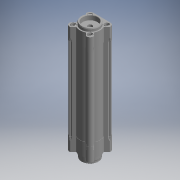
# Autodesk Inventor part: ESBF-BS-40-100---(ZR_-_-)
Saved by Autodesk Inventor 2017.3 (Build 213256000, 256)
## iProperties
Part Number: ESBF-BS-40-100---(ZR_-_-)
Material: Generic
Catalog Web Link: www.cadenas.de
Description: ESBF-(ZR)-Electro-cylinder
Vendor: FESTO
Document SubType Name: Modeling
Designer: partserver
Manufacturer: FESTO
Mass: 374.092 g
Surface Area: 1016.03 cm^2
Volume: 374.092 cm^3
Density: 1 g/cm^3
Appearance: PSOLRGB-192-192-192
Category: PARTsolutions
Company: FESTO
Title: ESBF-BS-40-100---(ZR_-_-)
Author: Cadenas PARTsolutions
Comments: Electro-cylinder
PSOL_IDENT_0: {$CADENAS_DATA\23d-libs\festo\parts\e\esbf\parts\esbf_zr.prj},208 {VTYP=3D},{NB=ESBF-BS-40-100---(ZR
PSOL_IDENT_1: _-_-)},{LINA=ESBF-BS-40-100---(ZR_-_-)},{NN=ESBF-(ZR)},{DATE=27.05.2021 13:20:18},{GEOMDATE=27.05.20
PSOL_IDENT_2: 21 13:19:59},{VERSION=},{LINEID=50},{WBVAR=HUB,SCEL,BWE},{WBNUMERIC=HUB}  {NB=ESBF-BS-40-100---(ZR_-
PSOL_IDENT_3: _-)},{LINA=ESBF-BS-40-100---(ZR_-_-)},{KT=DUMMY},{TNR=8022585},{TYP=ESBF-BS-40},{KDM=40},{HUB=100},{
PSOL_IDENT_4: SCEL=-},{BWE=-},{A=-6.000},{ANG=40.000},{B=39.000},{B1=38.000},{BE1=10.000},{BG=16.000},{D1=24.000},
PSOL_IDENT_5: {D2=8.000},{D2R=9.000},{D3=40.000},{D3R=10.500},{D5=33.000},{E=54.000},{E1=0.000},{EG=11.500},{G=30.
PSOL_IDENT_6: 000},{G1=30.000},{HE=2.100},{R1=8.000},{R1I=7.500},{R2=45.300},{TG=38.000},{RI=22.250},{RK=1.800},{T
PSOL_IDENT_7: 5=10.200},{J2=0.000},{L10=13.000},{L14=21.100},{L16=18.700},{L18=5.500},{L1=14.000},{L2=144.000},{L3=
PSOL_IDENT_8: 18.400},{L7=24.000},{M1=6.000},{PL=0.000},{SW3=6.000},{SWT=4.000},{VA=7.000},{VD=9.000},{D100=7.000}
PSOL_IDENT_9: ,{GUA=10.000},{B2=4.000},{D6=25.500},{D7=35.200},{BWE1='-','F1A'}
NB: ESBF-BS-40-100---(ZR_-_-)
NN: ESBF-(ZR)
NT: Electro-cylinder
NBSYN: $TYP.-$HUB.---(ZR_$SCEL._$BWE.)
LINA: ESBF-BS-40-100---(ZR_-_-)
CATALOG: Festo
TNR: 8022585
TYP: ESBF-BS-40
KDM: 40
HUB: 100
SCEL: -
BWE: -
A: -6
ANG: 40
B: 39
B1: 38
BE1: 10
BG: 16
D1: 24
D2: 8
D2R: 9
D3: 40
D3R: 10.5
D5: 33
E: 54
E1: 0
EG: 11.5
G: 30
G1: 30
HE: 2.1
R1: 8
R1I: 7.5
R2: 45.3
TG: 38
RI: 22.25
RK: 1.8
T5: 10.2
J2: 0
L10: 13
L14: 21.1
L16: 18.7
L18: 5.5
L1: 14
L2: 144
L3: 18.4
L7: 24
M1: 6
PL: 0
SW3: 6
SWT: 4
VA: 7
VD: 9
D100: 7
GUA: 10
B2: 4
D6: 25.5
D7: 35.2
SUPPLIER: FESTO
ARTICLENO: ESBF-BS-40-100---(ZR_-_-)
BOMINFO: ESBF-BS-40-100---(ZR_-_-)
CREATOR: CADENAS GmbH
Autodesk Inventor part; units mm, degrees
sketch "Sketch_1" plane through (0, 0, -30) normal (0, 0, 1) x (1, 0, 0)
  arc A0 (-27, 18.2218) -> (-26.7071, 17.5147) centre (-26, 18.2218) ccw
  line L0 (-26.7071, 17.5147) -> (-20.4561, 11.2637)
  arc A1 (-20.2683, 10.1102) -> (-20.4561, 11.2637) centre (-21.1632, 10.5566) ccw
  arc A2 (-20.2683, 10.1102) -> (-20.2683, -10.1102) centre (0, 0) ccw
  arc A3 (-20.4561, -11.2637) -> (-20.2683, -10.1102) centre (-21.1632, -10.5566) ccw
  line L1 (-20.4561, -11.2637) -> (-26.7071, -17.5147)
  arc A4 (-26.7071, -17.5147) -> (-27, -18.2218) centre (-26, -18.2218) ccw
  line L2 (-27, -18.2218) -> (-27, -19)
  arc A5 (-27, -19) -> (-19, -27) centre (-19, -19) ccw
  line L3 (-19, -27) -> (-18.2218, -27)
  arc A6 (-18.2218, -27) -> (-17.5147, -26.7071) centre (-18.2218, -26) ccw
  line L4 (-17.5147, -26.7071) -> (-11.2637, -20.4561)
  arc A7 (-10.1102, -20.2683) -> (-11.2637, -20.4561) centre (-10.5566, -21.1632) ccw
  arc A8 (-10.1102, -20.2683) -> (10.1102, -20.2683) centre (0, 0) ccw
  arc A9 (11.2637, -20.4561) -> (10.1102, -20.2683) centre (10.5566, -21.1632) ccw
  line L5 (11.2637, -20.4561) -> (17.5147, -26.7071)
  arc A10 (17.5147, -26.7071) -> (18.2218, -27) centre (18.2218, -26) ccw
  line L6 (18.2218, -27) -> (19, -27)
  arc A11 (19, -27) -> (27, -19) centre (19, -19) ccw
  line L7 (27, -19) -> (27, -18.2218)
  arc A12 (27, -18.2218) -> (26.7071, -17.5147) centre (26, -18.2218) ccw
  line L8 (26.7071, -17.5147) -> (20.4561, -11.2637)
  arc A13 (20.2683, -10.1102) -> (20.4561, -11.2637) centre (21.1632, -10.5566) ccw
  arc A14 (20.2683, -10.1102) -> (20.2683, 10.1102) centre (0, 0) ccw
  arc A15 (20.4561, 11.2637) -> (20.2683, 10.1102) centre (21.1632, 10.5566) ccw
  line L9 (20.4561, 11.2637) -> (26.7071, 17.5147)
  arc A16 (26.7071, 17.5147) -> (27, 18.2218) centre (26, 18.2218) ccw
  line L10 (27, 18.2218) -> (27, 19)
  arc A17 (27, 19) -> (19, 27) centre (19, 19) ccw
  line L11 (19, 27) -> (-19, 27)
  arc A18 (-19, 27) -> (-27, 19) centre (-19, 19) ccw
  line L12 (-27, 19) -> (-27, 18.2218)
  constraints: 38 point on circle, 26 end point, 19 centre point
extrude "Extrusion1" add sketch "Sketch_1" along normal blind 30
sketch "Sketch_8" plane through (0, 0, -30) normal (0, 0, 1) x (1, 0, 0)
  line L0 (-50, 45) -> (50, 45)
  line L1 (-19.3, 33.75) -> (-19.3, 27)
  line L2 (-19.3, 27) -> (-18.203, 25.1)
  arc A0 (-18.203, 25.1) -> (-18.0298, 25) centre (-18.0298, 25.2) ccw
  line L3 (-18.0298, 25) -> (-17.3281, 25)
  arc A1 (-17.3281, 25) -> (-17.1867, 25.0586) centre (-17.3281, 25.2) ccw
  line L4 (-17.1867, 25.0586) -> (-15.2453, 27)
  line L5 (-15.2453, 27) -> (15.2453, 27)
  line L6 (15.2453, 27) -> (17.1867, 25.0586)
  arc A2 (17.1867, 25.0586) -> (17.3281, 25) centre (17.3281, 25.2) ccw
  line L7 (17.3281, 25) -> (18.0298, 25)
  arc A3 (18.0298, 25) -> (18.203, 25.1) centre (18.0298, 25.2) ccw
  line L8 (18.203, 25.1) -> (19.3, 27)
  line L9 (19.3, 27) -> (19.3, 33.75)
  line L10 (19.3, 33.75) -> (-19.3, 33.75)
  constraints: 22 end point, 8 point on circle, 4 centre point
revolve "Revolution1" cut sketch "Sketch_8" angle 360 about axis through (-50, 45, -30) along (-1, 0, 0)
sketch "Sketch_21" plane through (0, 0, -30) normal (0, 0, 1) x (1, 0, 0)
  line L0 (50, -45) -> (-50, -45)
  line L1 (-19.3, -33.75) -> (19.3, -33.75)
  line L2 (19.3, -33.75) -> (19.3, -27)
  line L3 (19.3, -27) -> (18.203, -25.1)
  arc A0 (18.203, -25.1) -> (18.0298, -25) centre (18.0298, -25.2) ccw
  line L4 (18.0298, -25) -> (5.7378, -25)
  arc A1 (-5.7378, -25) -> (5.7378, -25) centre (0, 0) ccw
  line L5 (-5.7378, -25) -> (-18.0298, -25)
  arc A2 (-18.0298, -25) -> (-18.203, -25.1) centre (-18.0298, -25.2) ccw
  line L6 (-18.203, -25.1) -> (-19.3, -27)
  line L7 (-19.3, -27) -> (-19.3, -33.75)
  constraints: 16 end point, 6 point on circle, 3 centre point
revolve "Revolution2" cut sketch "Sketch_21" angle 360 about axis through (50, -45, -30) along (1, 0, 0)
sketch "Sketch_23" plane through (0, 0, -30) normal (0, 0, 1) x (1, 0, 0)
  line L0 (45, 50) -> (45, -50)
  line L1 (25, -5.7378) -> (25, -18.0298)
  arc A0 (25, -18.0298) -> (25.1, -18.203) centre (25.2, -18.0298) ccw
  line L2 (25.1, -18.203) -> (27, -19.3)
  line L3 (27, -19.3) -> (33.75, -19.3)
  line L4 (33.75, -19.3) -> (33.75, 19.3)
  line L5 (33.75, 19.3) -> (27, 19.3)
  line L6 (27, 19.3) -> (25.1, 18.203)
  arc A1 (25.1, 18.203) -> (25, 18.0298) centre (25.2, 18.0298) ccw
  line L7 (25, 18.0298) -> (25, 5.7378)
  arc A2 (25, -5.7378) -> (25, 5.7378) centre (0, 0) ccw
  constraints: 16 end point, 6 point on circle, 3 centre point
revolve "Revolution3" cut sketch "Sketch_23" angle 360 about axis through (45, 50, -30) along (0, 1, 0)
sketch "Sketch_24" plane through (0, 0, -30) normal (0, 0, 1) x (1, 0, 0)
  line L0 (-45, -50) -> (-45, 50)
  line L1 (-33.75, -19.3) -> (-27, -19.3)
  line L2 (-27, -19.3) -> (-25.1, -18.203)
  arc A0 (-25.1, -18.203) -> (-25, -18.0298) centre (-25.2, -18.0298) ccw
  line L3 (-25, -18.0298) -> (-25, -5.7378)
  arc A1 (-25, 5.7378) -> (-25, -5.7378) centre (0, 0) ccw
  line L4 (-25, 5.7378) -> (-25, 18.0298)
  arc A2 (-25, 18.0298) -> (-25.1, 18.203) centre (-25.2, 18.0298) ccw
  line L5 (-25.1, 18.203) -> (-27, 19.3)
  line L6 (-27, 19.3) -> (-33.75, 19.3)
  line L7 (-33.75, 19.3) -> (-33.75, -19.3)
  constraints: 16 end point, 6 point on circle, 3 centre point
revolve "Revolution4" cut sketch "Sketch_24" angle 360 about axis through (-45, -50, -30) along (0, -1, 0)
sketch "Sketch_41" plane through (0, 0, 0) normal (1, 0, 0) x (0, 1, 0)
  line L0 (0, -214) -> (0, -30)
  line L1 (0, -30) -> (5, -30)
  line L2 (5, -30) -> (5, -214)
  line L3 (5, -214) -> (0, -214)
  line L4 (0, -214) -> (0, -30)
  constraints: 10 end point
revolve "Revolution5" add sketch "Sketch_41" angle 360 about axis through (0, 0, -214) along (0, 0, -1)
sketch "Sketch_5" plane through (0, 0, -214) normal (0, 0, 1) x (1, 0, 0)
  arc A0 (-27, 18.2218) -> (-26.7071, 17.5147) centre (-26, 18.2218) ccw
  line L0 (-26.7071, 17.5147) -> (-20.4561, 11.2637)
  arc A1 (-20.2683, 10.1102) -> (-20.4561, 11.2637) centre (-21.1632, 10.5566) ccw
  arc A2 (-20.2683, 10.1102) -> (-20.2683, -10.1102) centre (0, 0) ccw
  arc A3 (-20.4561, -11.2637) -> (-20.2683, -10.1102) centre (-21.1632, -10.5566) ccw
  line L1 (-20.4561, -11.2637) -> (-26.7071, -17.5147)
  arc A4 (-26.7071, -17.5147) -> (-27, -18.2218) centre (-26, -18.2218) ccw
  line L2 (-27, -18.2218) -> (-27, -19)
  arc A5 (-27, -19) -> (-19, -27) centre (-19, -19) ccw
  line L3 (-19, -27) -> (-18.2218, -27)
  arc A6 (-18.2218, -27) -> (-17.5147, -26.7071) centre (-18.2218, -26) ccw
  line L4 (-17.5147, -26.7071) -> (-11.2637, -20.4561)
  arc A7 (-10.1102, -20.2683) -> (-11.2637, -20.4561) centre (-10.5566, -21.1632) ccw
  arc A8 (-10.1102, -20.2683) -> (10.1102, -20.2683) centre (0, 0) ccw
  arc A9 (11.2637, -20.4561) -> (10.1102, -20.2683) centre (10.5566, -21.1632) ccw
  line L5 (11.2637, -20.4561) -> (17.5147, -26.7071)
  arc A10 (17.5147, -26.7071) -> (18.2218, -27) centre (18.2218, -26) ccw
  line L6 (18.2218, -27) -> (19, -27)
  arc A11 (19, -27) -> (27, -19) centre (19, -19) ccw
  line L7 (27, -19) -> (27, -18.2218)
  arc A12 (27, -18.2218) -> (26.7071, -17.5147) centre (26, -18.2218) ccw
  line L8 (26.7071, -17.5147) -> (20.4561, -11.2637)
  arc A13 (20.2683, -10.1102) -> (20.4561, -11.2637) centre (21.1632, -10.5566) ccw
  arc A14 (20.2683, -10.1102) -> (20.2683, 10.1102) centre (0, 0) ccw
  arc A15 (20.4561, 11.2637) -> (20.2683, 10.1102) centre (21.1632, 10.5566) ccw
  line L9 (20.4561, 11.2637) -> (26.7071, 17.5147)
  arc A16 (26.7071, 17.5147) -> (27, 18.2218) centre (26, 18.2218) ccw
  line L10 (27, 18.2218) -> (27, 19)
  arc A17 (27, 19) -> (19, 27) centre (19, 19) ccw
  line L11 (19, 27) -> (-19, 27)
  arc A18 (-19, 27) -> (-27, 19) centre (-19, 19) ccw
  line L12 (-27, 19) -> (-27, 18.2218)
  constraints: 38 point on circle, 26 end point, 19 centre point
extrude "Extrusion2" add sketch "Sketch_5" against normal blind 30
sketch "Sketch_4" plane through (0, 0, -214) normal (0, 0, 1) x (1, 0, 0)
  line L0 (-50, 45) -> (50, 45)
  line L1 (-19.3, 33.75) -> (-19.3, 27)
  line L2 (-19.3, 27) -> (-18.203, 25.1)
  arc A0 (-18.203, 25.1) -> (-18.0298, 25) centre (-18.0298, 25.2) ccw
  line L3 (-18.0298, 25) -> (-17.3281, 25)
  arc A1 (-17.3281, 25) -> (-17.1867, 25.0586) centre (-17.3281, 25.2) ccw
  line L4 (-17.1867, 25.0586) -> (-15.2453, 27)
  line L5 (-15.2453, 27) -> (15.2453, 27)
  line L6 (15.2453, 27) -> (17.1867, 25.0586)
  arc A2 (17.1867, 25.0586) -> (17.3281, 25) centre (17.3281, 25.2) ccw
  line L7 (17.3281, 25) -> (18.0298, 25)
  arc A3 (18.0298, 25) -> (18.203, 25.1) centre (18.0298, 25.2) ccw
  line L8 (18.203, 25.1) -> (19.3, 27)
  line L9 (19.3, 27) -> (19.3, 33.75)
  line L10 (19.3, 33.75) -> (-19.3, 33.75)
  constraints: 22 end point, 8 point on circle, 4 centre point
revolve "Revolution6" cut sketch "Sketch_4" angle 360 about axis through (-50, 45, -214) along (-1, 0, 0)
sketch "Sketch_25" plane through (0, 0, -214) normal (0, 0, 1) x (1, 0, 0)
  line L0 (50, -45) -> (-50, -45)
  line L1 (-19.3, -27) -> (-19.3, -36)
  line L2 (-19.3, -36) -> (19.3, -36)
  line L3 (19.3, -36) -> (19.3, -27)
  line L4 (19.3, -27) -> (18.203, -25.1)
  arc A0 (18.203, -25.1) -> (18.0298, -25) centre (18.0298, -25.2) ccw
  line L5 (18.0298, -25) -> (5.7378, -25)
  arc A1 (-5.7378, -25) -> (5.7378, -25) centre (0, 0) ccw
  line L6 (-5.7378, -25) -> (-18.0298, -25)
  arc A2 (-18.0298, -25) -> (-18.203, -25.1) centre (-18.0298, -25.2) ccw
  line L7 (-18.203, -25.1) -> (-19.3, -27)
  constraints: 16 end point, 6 point on circle, 3 centre point
revolve "Revolution7" cut sketch "Sketch_25" angle 360 about axis through (50, -45, -214) along (1, 0, 0)
sketch "Sketch_26" plane through (0, 0, -214) normal (0, 0, 1) x (1, 0, 0)
  line L0 (45, 50) -> (45, -50)
  line L1 (25, -5.7378) -> (25, -18.0298)
  arc A0 (25, -18.0298) -> (25.1, -18.203) centre (25.2, -18.0298) ccw
  line L2 (25.1, -18.203) -> (27, -19.3)
  line L3 (27, -19.3) -> (33.75, -19.3)
  line L4 (33.75, -19.3) -> (33.75, 19.3)
  line L5 (33.75, 19.3) -> (27, 19.3)
  line L6 (27, 19.3) -> (25.1, 18.203)
  arc A1 (25.1, 18.203) -> (25, 18.0298) centre (25.2, 18.0298) ccw
  line L7 (25, 18.0298) -> (25, 5.7378)
  arc A2 (25, -5.7378) -> (25, 5.7378) centre (0, 0) ccw
  constraints: 16 end point, 6 point on circle, 3 centre point
revolve "Revolution8" cut sketch "Sketch_26" angle 360 about axis through (45, 50, -214) along (0, 1, 0)
sketch "Sketch_27" plane through (0, 0, -214) normal (0, 0, 1) x (1, 0, 0)
  line L0 (-45, -50) -> (-45, 50)
  line L1 (-33.75, -19.3) -> (-27, -19.3)
  line L2 (-27, -19.3) -> (-25.1, -18.203)
  arc A0 (-25.1, -18.203) -> (-25, -18.0298) centre (-25.2, -18.0298) ccw
  line L3 (-25, -18.0298) -> (-25, -5.7378)
  arc A1 (-25, 5.7378) -> (-25, -5.7378) centre (0, 0) ccw
  line L4 (-25, 5.7378) -> (-25, 18.0298)
  arc A2 (-25, 18.0298) -> (-25.1, 18.203) centre (-25.2, 18.0298) ccw
  line L5 (-25.1, 18.203) -> (-27, 19.3)
  line L6 (-27, 19.3) -> (-33.75, 19.3)
  line L7 (-33.75, 19.3) -> (-33.75, -19.3)
  constraints: 16 end point, 6 point on circle, 3 centre point
revolve "Revolution9" cut sketch "Sketch_27" angle 360 about axis through (-45, -50, -214) along (0, -1, 0)
sketch "Sketch_43" plane through (0, 0, -30) normal (0, 0, 1) x (1, 0, 0)
  arc A0 (-26.5208, -19.5466) -> (-26.7192, -19.9293) centre (-26.3208, -19.893) ccw
  arc A1 (-26.7192, -19.9293) -> (-19.9293, -26.7192) centre (-19.25, -19.25) ccw
  arc A2 (-19.9293, -26.7192) -> (-19.5466, -26.5208) centre (-19.893, -26.3208) ccw
  line L0 (-19.5466, -26.5208) -> (-18.582, -24.85)
  arc A3 (-18.2356, -24.65) -> (-18.582, -24.85) centre (-18.2356, -25.05) ccw
  line L1 (-18.2356, -24.65) -> (-15.9769, -24.65)
  arc A4 (-15.9769, -24.65) -> (-15.694, -24.5328) centre (-15.9769, -24.25) ccw
  line L2 (-15.694, -24.5328) -> (-11.6056, -20.4444)
  arc A5 (-9.5594, -20.0918) -> (-11.6056, -20.4444) centre (-10.3328, -21.7172) ccw
  arc A6 (-9.5594, -20.0918) -> (9.5594, -20.0918) centre (0, 0) ccw
  arc A7 (11.6056, -20.4444) -> (9.5594, -20.0918) centre (10.3328, -21.7172) ccw
  line L3 (11.6056, -20.4444) -> (15.694, -24.5328)
  arc A8 (15.694, -24.5328) -> (15.9769, -24.65) centre (15.9769, -24.25) ccw
  line L4 (15.9769, -24.65) -> (18.2356, -24.65)
  arc A9 (18.582, -24.85) -> (18.2356, -24.65) centre (18.2356, -25.05) ccw
  line L5 (18.582, -24.85) -> (19.5466, -26.5208)
  arc A10 (19.5466, -26.5208) -> (19.9293, -26.7192) centre (19.893, -26.3208) ccw
  arc A11 (19.9293, -26.7192) -> (26.7192, -19.9293) centre (19.25, -19.25) ccw
  arc A12 (26.7192, -19.9293) -> (26.5208, -19.5466) centre (26.3208, -19.893) ccw
  line L6 (26.5208, -19.5466) -> (24.85, -18.582)
  arc A13 (24.65, -18.2356) -> (24.85, -18.582) centre (25.05, -18.2356) ccw
  line L7 (24.65, -18.2356) -> (24.65, -15.9769)
  arc A14 (24.65, -15.9769) -> (24.5328, -15.694) centre (24.25, -15.9769) ccw
  line L8 (24.5328, -15.694) -> (20.4444, -11.6056)
  arc A15 (20.0918, -9.5594) -> (20.4444, -11.6056) centre (21.7172, -10.3328) ccw
  arc A16 (20.0918, -9.5594) -> (19.5191, 10.6803) centre (0, 0) ccw
  line L9 (19.5191, 10.6803) -> (24.5328, 15.694)
  arc A17 (24.5328, 15.694) -> (24.65, 15.9769) centre (24.25, 15.9769) ccw
  line L10 (24.65, 15.9769) -> (24.65, 18.2356)
  arc A18 (24.85, 18.582) -> (24.65, 18.2356) centre (25.05, 18.2356) ccw
  line L11 (24.85, 18.582) -> (26.5208, 19.5466)
  arc A19 (26.5208, 19.5466) -> (26.7192, 19.9293) centre (26.3208, 19.893) ccw
  arc A20 (26.7192, 19.9293) -> (19.9293, 26.7192) centre (19.25, 19.25) ccw
  arc A21 (19.9293, 26.7192) -> (19.5466, 26.5208) centre (19.893, 26.3208) ccw
  line L12 (19.5466, 26.5208) -> (18.582, 24.85)
  arc A22 (18.2356, 24.65) -> (18.582, 24.85) centre (18.2356, 25.05) ccw
  line L13 (18.2356, 24.65) -> (17.9713, 24.65)
  arc A23 (16.9107, 25.0893) -> (17.9713, 24.65) centre (17.9713, 26.15) ccw
  line L14 (16.9107, 25.0893) -> (15.25, 26.75)
  line L15 (15.25, 26.75) -> (-15.25, 26.75)
  line L16 (-15.25, 26.75) -> (-16.9107, 25.0893)
  arc A24 (-17.9713, 24.65) -> (-16.9107, 25.0893) centre (-17.9713, 26.15) ccw
  line L17 (-17.9713, 24.65) -> (-18.2356, 24.65)
  arc A25 (-18.582, 24.85) -> (-18.2356, 24.65) centre (-18.2356, 25.05) ccw
  line L18 (-18.582, 24.85) -> (-19.5466, 26.5208)
  arc A26 (-19.5466, 26.5208) -> (-19.9293, 26.7192) centre (-19.893, 26.3208) ccw
  arc A27 (-19.9293, 26.7192) -> (-26.7192, 19.9293) centre (-19.25, 19.25) ccw
  arc A28 (-26.7192, 19.9293) -> (-26.5208, 19.5466) centre (-26.3208, 19.893) ccw
  line L19 (-26.5208, 19.5466) -> (-24.85, 18.582)
  arc A29 (-24.65, 18.2356) -> (-24.85, 18.582) centre (-25.05, 18.2356) ccw
  line L20 (-24.65, 18.2356) -> (-24.65, 15.9769)
  arc A30 (-24.65, 15.9769) -> (-24.5328, 15.694) centre (-24.25, 15.9769) ccw
  line L21 (-24.5328, 15.694) -> (-19.5191, 10.6803)
  arc A31 (-19.5191, 10.6803) -> (-20.0918, -9.5594) centre (0, 0) ccw
  arc A32 (-20.4444, -11.6056) -> (-20.0918, -9.5594) centre (-21.7172, -10.3328) ccw
  line L22 (-20.4444, -11.6056) -> (-24.5328, -15.694)
  arc A33 (-24.5328, -15.694) -> (-24.65, -15.9769) centre (-24.25, -15.9769) ccw
  line L23 (-24.65, -15.9769) -> (-24.65, -18.2356)
  arc A34 (-24.85, -18.582) -> (-24.65, -18.2356) centre (-25.05, -18.2356) ccw
  line L24 (-24.85, -18.582) -> (-26.5208, -19.5466)
  constraints: 70 point on circle, 50 end point, 35 centre point
extrude "Extrusion3" add sketch "Sketch_43" against normal blind 184
sketch "Sketch_3" plane through (0, 0, 0) normal (1, 0, 0) x (0, 1, 0)
  line L0 (0, 0) -> (0, 18)
  line L1 (0, 18) -> (12.75, 18)
  arc A0 (12.75, 18) -> (13.4103, 16.8683) centre (14.05, 18) ccw
  line L2 (13.4103, 16.8683) -> (17.6, 14.5)
  line L3 (17.6, 14.5) -> (17.6, 14)
  line L4 (17.6, 14) -> (18.5, 14)
  line L5 (18.5, 14) -> (19, 13.5)
  line L6 (19, 13.5) -> (19, 9.866)
  line L7 (19, 9.866) -> (19.5, 9)
  line L8 (19.5, 9) -> (19.5, 0)
  line L9 (19.5, 0) -> (0, 0)
  line L10 (0, 0) -> (0, 18)
  constraints: 22 end point, 2 point on circle, 1 centre point
revolve "Revolution10" add sketch "Sketch_3" angle 360 about axis through (0, 0, 0) along (0, 0, -1)
sketch "Sketch_40" plane through (0, 0, -220) normal (0, 0, 1) x (1, 0, 0)
  line L0 (0, 26.7) -> (0, 27)
  line L1 (0, 27) -> (5, 27)
  line L2 (5, 27) -> (5, 26.7)
  line L3 (5, 26.7) -> (0, 26.7)
  line L4 (0, 26.7) -> (0, 27)
  constraints: 10 end point
revolve "Revolution11" cut sketch "Sketch_40" angle 360 about axis through (0, 26.7, -220) along (0, -1, 0)
sketch "Sketch_9" plane through (19, 0, 0) normal (1, 0, 0) x (0, 0, -1)
  line L0 (21.1, 19) -> (0, 19)
  line L1 (0, 19) -> (0, 24.25)
  line L2 (0, 24.25) -> (21.1, 24.25)
  line L3 (21.1, 24.25) -> (21.1, 19)
  line L4 (21.1, 19) -> (0, 19)
  constraints: 10 end point
revolve "Revolution12" cut sketch "Sketch_9" angle 360 about axis through (19, 19, -21.1) along (0, 0, -1)
pattern_linear "Rectangular Pattern1" count 2 spacing 38 along (-1, 0, 0) count 2 spacing 38 along (0, -1, 0) of "Revolution12"
sketch "Sketch_11" plane through (19, 0, 0) normal (1, 0, 0) x (0, 0, -1)
  line L0 (21.1, 19) -> (0, 19)
  line L1 (0, 19) -> (0, 22.6609)
  line L2 (0, 22.6609) -> (1, 23.5)
  line L3 (1, 23.5) -> (21.1, 23.5)
  line L4 (21.1, 23.5) -> (21.1, 19)
  line L5 (21.1, 19) -> (0, 19)
  constraints: 12 end point
revolve "Revolution13" add sketch "Sketch_11" angle 360 about axis through (19, 19, -21.1) along (0, 0, -1)
pattern_linear "Rectangular Pattern2" count 2 spacing 38 along (-1, 0, 0) count 2 spacing 38 along (0, -1, 0) of "Revolution13"
sketch "Sketch_13" plane through (19, 0, 0) normal (1, 0, 0) x (0, 0, -1)
  line L0 (20.1194, 19) -> (0, 19)
  line L1 (0, 19) -> (0, 22.5)
  line L2 (0, 22.5) -> (0.2887, 22)
  line L3 (0.2887, 22) -> (5.5, 22)
  line L4 (5.5, 22) -> (6.0415, 21.4585)
  line L5 (6.0415, 21.4585) -> (18.7, 21.4585)
  line L6 (18.7, 21.4585) -> (20.1194, 19)
  line L7 (20.1194, 19) -> (0, 19)
  constraints: 16 end point
revolve "Revolution14" cut sketch "Sketch_13" angle 360 about axis through (19, 19, -20.1194) along (0, 0, -1)
thread "Thread1" size "M6x1" class "6H" standard "ISO Metric profile" length 9.9585
sketch "Sketch_14" plane through (0, 0, 0) normal (0, 0, 1) x (1, 0, 0)
  line L0 (15.5359, 19) -> (16, 18.1962)
  line L1 (16, 18.1962) -> (16, 17.2679)
  line L2 (16, 17.2679) -> (16.8038, 16.8038)
  line L3 (16.8038, 16.8038) -> (17.2679, 16)
  line L4 (17.2679, 16) -> (18.1962, 16)
  line L5 (18.1962, 16) -> (19, 15.5359)
  line L6 (19, 15.5359) -> (19.8038, 16)
  line L7 (19.8038, 16) -> (20.7321, 16)
  line L8 (20.7321, 16) -> (21.1962, 16.8038)
  line L9 (21.1962, 16.8038) -> (22, 17.2679)
  line L10 (22, 17.2679) -> (22, 18.1962)
  line L11 (22, 18.1962) -> (22.4641, 19)
  line L12 (22.4641, 19) -> (22, 19.8038)
  line L13 (22, 19.8038) -> (22, 20.7321)
  line L14 (22, 20.7321) -> (21.1962, 21.1962)
  line L15 (21.1962, 21.1962) -> (20.7321, 22)
  line L16 (20.7321, 22) -> (19.8038, 22)
  line L17 (19.8038, 22) -> (19, 22.4641)
  line L18 (19, 22.4641) -> (18.1962, 22)
  line L19 (18.1962, 22) -> (17.2679, 22)
  line L20 (17.2679, 22) -> (16.8038, 21.1962)
  line L21 (16.8038, 21.1962) -> (16, 20.7321)
  line L22 (16, 20.7321) -> (16, 19.8038)
  line L23 (16, 19.8038) -> (15.5359, 19)
  constraints: 48 end point
extrude "Extrusion4" cut sketch "Sketch_14" along normal mid plane 8
pattern_linear "Rectangular Pattern3" count 2 spacing 38 along (-1, 0, 0) count 2 spacing 38 along (0, -1, 0) of "Revolution14"
pattern_linear "Rectangular Pattern4" count 2 spacing 38 along (-1, 0, 0) count 2 spacing 38 along (0, -1, 0) of "Extrusion4"
sketch "Sketch_22" plane through (0, 0, 0) normal (1, 0, 0) x (0, 1, 0)
  line L0 (0, -251) -> (0, -244)
  line L1 (0, -244) -> (20, -244)
  line L2 (20, -244) -> (20, -249)
  line L3 (20, -249) -> (19.2721, -251)
  line L4 (19.2721, -251) -> (0, -251)
  line L5 (0, -251) -> (0, -244)
  constraints: 12 end point
revolve "Revolution15" add sketch "Sketch_22" angle 360 about axis through (0, 0, -251) along (0, 0, -1)
sketch "Sketch_2" plane through (0, 0, 0) normal (1, 0, 0) x (0, 1, 0)
  line L0 (0, -251) -> (0, -214)
  line L1 (0, -214) -> (5, -214)
  line L2 (5, -214) -> (5, -240.8)
  line L3 (5, -240.8) -> (16.5, -240.8)
  line L4 (16.5, -240.8) -> (16.5, -250)
  line L5 (16.5, -250) -> (16.864, -251)
  line L6 (16.864, -251) -> (0, -251)
  line L7 (0, -251) -> (0, -214)
  constraints: 16 end point
revolve "Revolution16" cut sketch "Sketch_2" angle 360 about axis through (0, 0, -251) along (0, 0, -1)
sketch "Sketch21" plane through (0, 0, -244) normal (0, 0, -1) x (-1, 0, 0)
  point P0 (-19, 19)
hole "Hole1" at (19, 19, -244) direction (0, 0, 1) diameter 10.5 depth 21.1
pattern_linear "Rectangular Pattern5" count 2 spacing 38 along (-1, 0, 0) count 2 spacing 38 along (0, -1, 0) of "Hole1"
sketch "Sketch_30" plane through (19, 0, 0) normal (1, 0, 0) x (0, 0, -1)
  line L0 (244, 19) -> (222.9, 19)
  line L1 (222.9, 19) -> (222.9, 23.5)
  line L2 (222.9, 23.5) -> (243, 23.5)
  line L3 (243, 23.5) -> (244, 22.6609)
  line L4 (244, 22.6609) -> (244, 19)
  line L5 (244, 19) -> (222.9, 19)
  constraints: 12 end point
revolve "Revolution17" add sketch "Sketch_30" angle 360 about axis through (19, 19, -244) along (0, 0, -1)
pattern_linear "Rectangular Pattern6" count 2 spacing 38 along (-1, 0, 0) count 2 spacing 38 along (0, -1, 0) of "Revolution17"
sketch "Sketch_32" plane through (19, 0, 0) normal (1, 0, 0) x (0, 0, -1)
  line L0 (244, 19) -> (223.8806, 19)
  line L1 (223.8806, 19) -> (225.3, 21.4585)
  line L2 (225.3, 21.4585) -> (237.9585, 21.4585)
  line L3 (237.9585, 21.4585) -> (238.5, 22)
  line L4 (238.5, 22) -> (243.7113, 22)
  line L5 (243.7113, 22) -> (244, 22.5)
  line L6 (244, 22.5) -> (244, 19)
  line L7 (244, 19) -> (223.8806, 19)
  constraints: 16 end point
revolve "Revolution18" cut sketch "Sketch_32" angle 360 about axis through (19, 19, -244) along (0, 0, -1)
thread "Thread2" size "M6x1" class "6H" standard "ISO Metric profile" length 9.9585
pattern_linear "Rectangular Pattern7" count 2 spacing 38 along (-1, 0, 0) count 2 spacing 38 along (0, -1, 0) of "Revolution18"
sketch "Sketch_34" plane through (0, 0, -244) normal (0, 0, 1) x (1, 0, 0)
  line L0 (15.5359, 19) -> (16, 18.1962)
  line L1 (16, 18.1962) -> (16, 17.2679)
  line L2 (16, 17.2679) -> (16.8038, 16.8038)
  line L3 (16.8038, 16.8038) -> (17.2679, 16)
  line L4 (17.2679, 16) -> (18.1962, 16)
  line L5 (18.1962, 16) -> (19, 15.5359)
  line L6 (19, 15.5359) -> (19.8038, 16)
  line L7 (19.8038, 16) -> (20.7321, 16)
  line L8 (20.7321, 16) -> (21.1962, 16.8038)
  line L9 (21.1962, 16.8038) -> (22, 17.2679)
  line L10 (22, 17.2679) -> (22, 18.1962)
  line L11 (22, 18.1962) -> (22.4641, 19)
  line L12 (22.4641, 19) -> (22, 19.8038)
  line L13 (22, 19.8038) -> (22, 20.7321)
  line L14 (22, 20.7321) -> (21.1962, 21.1962)
  line L15 (21.1962, 21.1962) -> (20.7321, 22)
  line L16 (20.7321, 22) -> (19.8038, 22)
  line L17 (19.8038, 22) -> (19, 22.4641)
  line L18 (19, 22.4641) -> (18.1962, 22)
  line L19 (18.1962, 22) -> (17.2679, 22)
  line L20 (17.2679, 22) -> (16.8038, 21.1962)
  line L21 (16.8038, 21.1962) -> (16, 20.7321)
  line L22 (16, 20.7321) -> (16, 19.8038)
  line L23 (16, 19.8038) -> (15.5359, 19)
  constraints: 48 end point
extrude "Extrusion5" cut sketch "Sketch_34" along normal mid plane 8
pattern_linear "Rectangular Pattern8" count 2 spacing 38 along (-1, 0, 0) count 2 spacing 38 along (0, -1, 0) of "Extrusion5"
sketch "Sketch25" plane through (0, 0, -214) normal (0, 0, -1) x (-1, 0, 0)
  point P0 (0, 0)
hole "Hole2" at (0, 0, -214) direction (0, 0, 1) diameter 24 depth 232 counterbore diameter 40 counterbore depth 113.3333
ref_plane "GUA_XY" through (0, 0, -240.8) normal (0, 0, 1) x (0, 1, 0)
ref_plane "GUA_YZ" through (0, 0, -240.8) normal (0, 1, 0) x (-1, 0, 0)
ref_plane "GUA_ZX" through (0, 0, -240.8) normal (-1, 0, 0) x (0, 0, 1)
ref_plane "KS_XY" through (0, 0, -214) normal (0, 0, 1) x (1, 0, 0)
ref_plane "KS_YZ" through (0, 0, -214) normal (1, 0, 0) x (0, 1, 0)
ref_plane "KS_ZX" through (0, 0, -214) normal (0, 1, 0) x (0, 0, 1)
ref_plane "KSA_XY" through (0, 0, -214) normal (0, 0, -1) x (1, 0, 0)
ref_plane "KSA_YZ" through (0, 0, -214) normal (1, 0, 0) x (0, -1, 0)
ref_plane "KSA_ZX" through (0, 0, -214) normal (0, -1, 0) x (0, 0, -1)
ref_plane "PLUG_XY" through (0, 27, -220) normal (0, -1, 0) x (1, 0, 0)
ref_plane "PLUG_YZ" through (0, 27, -220) normal (1, 0, 0) x (0, 0, 1)
ref_plane "PLUG_ZX" through (0, 27, -220) normal (0, 0, 1) x (0, -1, 0)
ref_plane "SENSOR_XY" through (0, 27, -122) normal (0, 0, 1) x (1, 0, 0)
ref_plane "SENSOR_YZ" through (0, 27, -122) normal (1, 0, 0) x (0, 1, 0)
ref_plane "SENSOR_ZX" through (0, 27, -122) normal (0, 1, 0) x (0, 0, 1)
ref_plane "START_XY" through (0, 0, 0) normal (0, 0, -1) x (1, 0, 0)
ref_plane "START_YZ" through (0, 0, 0) normal (1, 0, 0) x (0, -1, 0)
ref_plane "START_ZX" through (0, 0, 0) normal (0, -1, 0) x (0, 0, -1)
body "Solid1"
